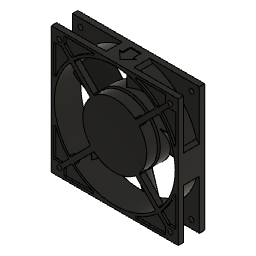
Fan 120mm (Autodesk Fusion 360 design; units mm, degrees)
Autodesk Fusion 360 part; units mm, degrees
sketch "Frame1" plane through (0, 0, 0) normal (0, 1, 0) x (1, 0, 0)
  line L0 (60, 60) -> (-60, 60)
  line L1 (-60, 60) -> (-60, -60)
  line L2 (-60, -60) -> (60, -60)
  line L3 (60, -60) -> (60, 60)
  line L4 (60, 60) -> (-60, -60) construction
  line L5 (-60, 60) -> (60, -60) construction
  circle A0 centre (0, 0) radius 57.125
  circle A1 centre (0, 0) radius 30.25
  circle A2 centre (-52.5, -52.5) radius 2.3
  line L6 (-65, 0) -> (65, 0) construction
  line L7 (0, -65) -> (0, 65) construction
  circle A3 centre (-52.5, 52.5) radius 2.3
  circle A4 centre (52.5, -52.5) radius 2.3
  circle A5 centre (52.5, 52.5) radius 2.3
  circle A6 centre (0, 0) radius 59.4
  line L8 (57.75, -57.75) -> (-57.75, -57.75)
  line L9 (-57.75, -57.75) -> (-57.75, 57.75)
  line L10 (-57.75, 57.75) -> (57.75, 57.75)
  line L11 (57.75, 57.75) -> (57.75, -57.75)
  line L12 (57.75, -57.75) -> (-57.75, 57.75) construction
  line L13 (-57.75, -57.75) -> (57.75, 57.75) construction
  line L14 (-60, -60) -> (-48, -60)
  line L15 (-48, -60) -> (-48, -48)
  line L16 (-48, -48) -> (-60, -48)
  line L17 (-60, -48) -> (-60, -60)
  line L18 (-48, 60) -> (-48, 48)
  line L19 (-48, 48) -> (-60, 48)
  line L20 (48, -60) -> (48, -48)
  line L21 (48, -48) -> (60, -48)
  line L22 (48, 48) -> (60, 48)
  line L23 (48, 60) -> (48, 48)
  line L24 (-9.1263, -5.8737) -> (5.8737, 9.1263) construction
  line L25 (2.5831, -0.6696) -> (-40.3443, -43.597) construction
  line L26 (-40.8339, -38.1469) -> (-47.3531, -44.6661) construction
  line L27 (-38.9044, -41.5914) -> (-49.6566, -52.3436) construction
  line L28 (-44, -38) -> (-38.4801, -43.5199) construction
  line L29 (-42.3435, -39.6565) -> (-39.6565, -42.3435)
  line L30 (-39.6565, -42.3435) -> (-48.8653, -51.5523)
  line L31 (-48.8653, -51.5523) -> (-51.5523, -48.8653)
  line L32 (-51.5523, -48.8653) -> (-42.3435, -39.6565)
  line L33 (-39.6565, 42.3435) -> (-48.8653, 51.5523)
  line L34 (-51.5523, 48.8653) -> (-42.3435, 39.6565)
  line L35 (51.5523, -48.8653) -> (42.3435, -39.6565)
  line L36 (39.6565, -42.3435) -> (48.8653, -51.5523)
  line L37 (51.5523, 48.8653) -> (42.3435, 39.6565)
  line L38 (39.6565, 42.3435) -> (48.8653, 51.5523)
  line L39 (-1.6263, 1.6263) -> (1.6263, -1.6263)
  line L40 (1.6263, -1.6263) -> (-39.0908, -42.3435)
  line L41 (-39.0908, -42.3435) -> (-42.3435, -39.0908)
  line L42 (-42.3435, -39.0908) -> (-1.6263, 1.6263)
  line L43 (1.6263, 1.6263) -> (-39.0908, 42.3435)
  line L44 (-42.3435, 39.0908) -> (-1.6263, -1.6263)
  line L45 (42.3435, 39.0908) -> (1.6263, -1.6263)
  line L46 (-1.6263, 1.6263) -> (39.0908, 42.3435)
  line L47 (42.3435, -39.0908) -> (1.6263, 1.6263)
  line L48 (-1.6263, -1.6263) -> (39.0908, -42.3435)
  dimension "d1" = 120
  dimension "d2" = 120
  dimension "d3" = 114.25
  dimension "d4" = 60.5
  dimension "d5" = 4.6
  dimension "d6" = 7.5
  dimension "d7" = 118.8
  dimension "d8" = 115.5
  dimension "d9" = 115.5
  dimension "d10" = 12
  dimension "d11" = 12
  dimension "d12" = 2.3
  dimension "d13" = 2.3
  dimension "d14" = 1.9
  dimension "d15" = 1.9
  constraint perpendicular L0 L1
  constraint parallel L0 L2
  constraint parallel L1 L3
  constraint horizontal L0
  constraint coincident L4 A0.centre
  constraint coincident L5 A0.centre
  constraint coincident A0.centre A1.centre
  constraint concentric A0 A1
  constraint coincident L4 A2.centre
  constraint perpendicular L3 L6
  constraint perpendicular L0 L7
  constraint symmetric A2 L6 A3
  constraint symmetric A2 L7 A4
  constraint symmetric L7 A3 A5
  constraint perpendicular L8 L9
  constraint parallel L8 L10
  constraint parallel L9 L11
  constraint horizontal L8
  constraint coincident L12 A0.centre
  constraint coincident L13 A0.centre
  constraint horizontal L14
  constraint vertical L15
  constraint horizontal L16
  constraint vertical L17
  constraint symmetric L6 L14.end L18.start
  constraint symmetric L6 L15.end L18.end
  constraint symmetric L6 L16.end L19.end
  constraint symmetric L7 L14.end L20.start
  constraint symmetric L7 L15.end L20.end
  constraint symmetric L7 L16.end L21.end
  constraint symmetric L7 L18.start L23.start
  constraint symmetric L7 L18.end L22.start
  constraint symmetric L7 L19.end L22.end
  constraint perpendicular L12 L24
  constraint coincident A6 L25.end
  constraint parallel L4 L25
  constraint parallel L13 L26
  constraint parallel L13 L27
  constraint perpendicular L25 L28
  constraint perpendicular L29 L30
  constraint parallel L29 L31
  constraint parallel L30 L32
  constraint coincident L28 L29.end
  constraint coincident L27 L29.end
  constraint perpendicular L27 L29
  constraint coincident L26 L29.start
  constraint symmetric L6 L29.start L34.end
  constraint symmetric L6 L29.end L33.start
  constraint symmetric L6 L30.end L33.end
  constraint symmetric L6 L31.end L34.start
  constraint symmetric L7 L29.start L35.end
  constraint symmetric L7 L29.end L36.start
  constraint symmetric L7 L30.end L36.end
  constraint symmetric L7 L31.end L35.start
  constraint symmetric L7 L33.start L38.start
  constraint symmetric L7 L33.end L38.end
  constraint symmetric L7 L34.start L37.start
  constraint symmetric L7 L34.end L37.end
  constraint perpendicular L39 L40
  constraint parallel L39 L41
  constraint parallel L40 L42
  constraint coincident L25 L39.end
  constraint coincident L5 L39.end
  constraint midpoint L24 L39.start
  constraint symmetric L6 L39.start L44.end
  constraint symmetric L6 L39.end L43.start
  constraint symmetric L6 L40.end L43.end
  constraint symmetric L6 L41.end L44.start
  constraint symmetric L7 L39.start L43.start
  constraint symmetric L7 L39.end L44.end
  constraint symmetric L7 L40.end L48.end
  constraint symmetric L7 L41.end L47.start
  constraint symmetric L7 L43.start L39.start
  constraint symmetric L7 L43.end L46.end
  constraint symmetric L7 L44.start L45.start
  constraint symmetric L7 L44.end L39.end
  measures "d1" distance of L1.end L2.end
  measures "d2" distance of L0.end L1.end
  measures "d3" diameter of A0
  measures "d4" diameter of A1
  measures "d5" diameter of A2
  measures "d6" distance of L1 A2.centre
  measures "d7" diameter of A6
  measures "d8" distance of L9.end L10.end
  measures "d9" distance of L8.end L9.end
  measures "d10" distance of L1.end L14.end
  measures "d11" distance of L1.end L16.end
  measures "d12" distance of L4 L24
  measures "d13" distance of L13 L25
  measures "d14" distance of L4 L26
  measures "d15" distance of L4 L27
  measures "d49" diameter of L0.start
extrude "Extrude1" add sketch "Frame1" against normal blind 5 from surface at -7.5 contours L0 L3 L10 L11 L22 L23 | L0 A6 L10 L18 L23 | L3 A6 L11 L21 L22 | L0 L1 L9 L10 L18 L19 | L10 L11 L22 L23 | L2 L3 L8 L11 L20 L21 | L9 L10 L18 L19 | A6 L10 | A6 L8 L9 L10 L11 L29 L30 L32 | A6 L22 L23 L37 L38 | L8 L11 L20 L21 | A6 L11 | L1 A6 L9 L16 L19 | A6 L18 L19 L33 L34 | L2 A6 L8 L15 L20 | A6 L20 L21 L35 L36 | L1 L2 L8 L9 L14 L15 L16 L17 | L8 L9 L15 L16 L30 L31 L32 | A6 L9 | A6 L8 | A6 L15 L16 L30 L32 | L15 L16 L30 L31 L32 | A6 L29 L30 L32 | A0 A1 L45 L46 | A0 A1 L47 L48 | A1 L43 L45 L46 L47 | A1 L45 L47 | A1 L40 L45 L47 L48 | A0 A1 L43 L44 | A1 L43 L46 | L39 L43 L45 L46 L47 | A0 L40 L41 L42 | A0 A1 L40 L42 | A1 L40 L48 | A1 L42 L43 L44 L46 | L39 L40 L42 L44 L48 | A1 L40 L42 L44 L48 | A1 L42 L44 makes body 1
extrude "Extrude2" add sketch "Frame1" along normal blind 5 from surface at 7.5 separate body contours L0 L3 L10 L11 L22 L23 | L0 A6 L10 L18 L23 | L3 A6 L11 L21 L22 | L0 L1 L9 L10 L18 L19 | L10 L11 L22 L23 | L2 L3 L8 L11 L20 L21 | L9 L10 L18 L19 | A6 L10 | A6 L8 L9 L10 L11 L29 L30 L32 | A6 L22 L23 L37 L38 | L8 L11 L20 L21 | A6 L11 | L1 A6 L9 L16 L19 | A6 L18 L19 L33 L34 | L2 A6 L8 L15 L20 | A6 L20 L21 L35 L36 | L1 L2 L8 L9 L14 L15 L16 L17 | L8 L9 L15 L16 L30 L31 L32 | A6 L9 | A6 L8 | A6 L15 L16 L30 L32 | L15 L16 L30 L31 L32 | A6 L29 L30 L32 | A0 L40 L41 L42 makes body 2
fillet "Fillet1" radius 1 32 edges at (13.9031, 10, 57.75) (-13.9031, 10, 57.75) (-48, 10, 57.75) (-48, 10, 50.687) (-40.6371, 10, 43.3242) (48, 10, 57.75) (48, 10, 50.687) (40.6371, 10, 43.3242) (43.3242, 10, 40.6371) (50.687, 10, 48) (57.75, 10, 48) (57.75, 10, 13.9031) (57.75, 10, -13.9031) (43.3242, 10, -40.6371) (50.687, 10, -48) (57.75, 10, -48) (40.6371, 10, -43.3242) (48, 10, -50.687) (48, 10, -57.75) (13.9031, 10, -57.75) (-13.9031, 10, -57.75) (-48, 10, -57.75) (-48, 10, -50.687) (-40.6371, 10, -43.3242) (-43.3242, 10, -40.6371) (-50.687, 10, -48) (-57.75, 10, -48) (-57.75, 10, -13.9031) (-57.75, 10, 13.9031) (-57.75, 10, 48) (-50.687, 10, 48) (-43.3242, 10, 40.6371) on bodies 2
extrude "Extrude3" add sketch "Frame1" against normal blind 3 from surface at -7.5 contours A6 L10 L23 L38 | A6 L11 L22 L37 | A6 L10 L18 L33 | A6 L11 L21 L35 | A6 L9 L19 L34 | A6 L8 L20 L36 | A6 L9 L16 L32 | A6 L8 L15 L30 bodies 1
extrude "Extrude4" add sketch "Frame1" along normal blind 3 from surface at 7.5 contours A6 L10 L23 L38 | A6 L11 L22 L37 | A6 L10 L18 L33 | A6 L11 L21 L35 | A6 L9 L19 L34 | A6 L8 L20 L36 | A6 L9 L16 L32 | A6 L8 L15 L30 bodies 2
extrude "Extrude5" add sketch "Frame1" against normal blind 5 from surface at -2.5 contours A1 L43 L45 L46 L47 | A1 L45 L47 | A1 L40 L45 L47 L48 | A1 L43 L46 | L39 L43 L45 L46 L47 | A1 L40 L48 | A1 L42 L43 L44 L46 | L39 L40 L42 L44 L48 | A1 L40 L42 L44 L48 | A1 L42 L44 bodies 1
fillet "Fillet2" radius 1 52 edges at (13.9031, -11.5, 57.75) (48, -11.5, 57.75) (40.6371, -11.5, 43.3242) (48, -11.5, 50.687) (43.3242, -11.5, 40.6371) (50.687, -11.5, 48) (57.75, -11.5, 48) (57.75, -11.5, 13.9031) (57.75, -11.5, -13.9031) (43.3242, -11.5, -40.6371) (50.687, -11.5, -48) (57.75, -11.5, -48) (40.6371, -11.5, -43.3242) (48, -11.5, -50.687) (48, -11.5, -57.75) (13.9031, -11.5, -57.75) (-13.9031, -11.5, -57.75) (-48, -11.5, -57.75) (-48, -11.5, -50.687) (-40.6371, -11.5, -43.3242) (-43.3242, -11.5, -40.6371) (-50.687, -11.5, -48) (-57.75, -11.5, -48) (-57.75, -11.5, -13.9031) (-57.75, -11.5, 13.9031) (-43.3242, -11.5, 40.6371) (-50.687, -11.5, 48) (-57.75, -11.5, 48) (-40.6371, -11.5, 43.3242) (-48, -11.5, 50.687) (-48, -11.5, 57.75) (-13.9031, -11.5, 57.75) (38.7344, -10, 41.9871) (19.7017, -10, 22.9544) (22.9544, -10, 19.7017) (41.9871, -10, 38.7344) (-38.7344, -10, 41.9871) (-41.9871, -10, 38.7344) (-22.9544, -10, 19.7017) (-19.7017, -10, 22.9544) (-22.9544, -10, -19.7017) (-19.7017, -10, -22.9544) (-41.9871, -10, -38.7344) (-38.7344, -10, -41.9871) (38.7344, -10, -41.9871) (41.9871, -10, -38.7344) (22.9544, -10, -19.7017) (19.7017, -10, -22.9544) (-21.39, -7.5, -21.39) (-21.39, -7.5, 21.39) (21.39, -7.5, 21.39) (21.39, -7.5, -21.39) on bodies 1
sketch "Frame2" plane through (0, -7.5, 0) normal (0, 1, 0) x (-1, 0, 0)
  line L0 (60, -60) -> (60, 60)
  line L1 (60, 60) -> (-60, 60)
  line L2 (-60, 60) -> (-60, -60)
  line L3 (-60, -60) -> (60, -60)
  circle A0 centre (-52.5, -52.5) radius 2.3
  arc A1 (-23.6635, -20.4108) -> (-20.4108, -23.6635) centre (0, 0) ccw
  line L4 (-23.6635, -20.4108) -> (-41.2441, -37.9914)
  arc A2 (-42.6986, -37.9486) -> (-41.2441, -37.9914) centre (-41.9512, -37.2843) ccw
  arc A3 (-42.6986, 37.9486) -> (-42.6986, -37.9486) centre (0, 0) ccw
  arc A4 (-41.2441, 37.9914) -> (-42.6986, 37.9486) centre (-41.9512, 37.2843) ccw
  line L5 (-41.2441, 37.9914) -> (-23.6635, 20.4108)
  arc A5 (-20.4108, 23.6635) -> (-23.6635, 20.4108) centre (0, 0) ccw
  line L6 (-20.4108, 23.6635) -> (-37.9914, 41.2441)
  arc A6 (-37.9486, 42.6986) -> (-37.9914, 41.2441) centre (-37.2843, 41.9512) ccw
  arc A7 (37.9486, 42.6986) -> (-37.9486, 42.6986) centre (0, 0) ccw
  arc A8 (37.9914, 41.2441) -> (37.9486, 42.6986) centre (37.2843, 41.9512) ccw
  line L7 (37.9914, 41.2441) -> (20.4108, 23.6635)
  arc A9 (23.6635, 20.4108) -> (20.4108, 23.6635) centre (0, 0) ccw
  line L8 (23.6635, 20.4108) -> (41.2441, 37.9914)
  arc A10 (42.6986, 37.9486) -> (41.2441, 37.9914) centre (41.9512, 37.2843) ccw
  arc A11 (42.6986, -37.9486) -> (42.6986, 37.9486) centre (0, 0) ccw
  arc A12 (41.2441, -37.9914) -> (42.6986, -37.9486) centre (41.9512, -37.2843) ccw
  line L9 (41.2441, -37.9914) -> (23.6635, -20.4108)
  arc A13 (20.4108, -23.6635) -> (23.6635, -20.4108) centre (0, 0) ccw
  line L10 (20.4108, -23.6635) -> (37.9914, -41.2441)
  arc A14 (37.9486, -42.6986) -> (37.9914, -41.2441) centre (37.2843, -41.9512) ccw
  arc A15 (-37.9486, -42.6986) -> (37.9486, -42.6986) centre (0, 0) ccw
  arc A16 (-37.9914, -41.2441) -> (-37.9486, -42.6986) centre (-37.2843, -41.9512) ccw
  line L11 (-37.9914, -41.2441) -> (-20.4108, -23.6635)
  circle A17 centre (52.5, 52.5) radius 2.3
  circle A18 centre (52.5, -52.5) radius 2.3
  circle A19 centre (-52.5, 52.5) radius 2.3
  circle A20 centre (0, 0) radius 57.125
  circle A21 centre (0, 0) radius 59.4
  line L12 (-60, -16) -> (-60, 16)
  line L13 (60, 16) -> (60, -16)
  line L14 (60, -16) -> (-60, 16) construction
  line L15 (-60, -16) -> (60, 16) construction
  line L16 (16, 60) -> (-16, 60)
  line L17 (-16, -60) -> (16, -60)
  line L18 (16, 60) -> (-16, -60) construction
  line L19 (-16, 60) -> (16, -60) construction
  line L20 (16, 57.2045) -> (16, 60)
  line L21 (-16, 60) -> (-16, 57.2045)
  line L22 (-16, -57.2045) -> (-16, -60)
  line L23 (57.2045, 16) -> (60, 16)
  line L24 (60, -16) -> (57.2045, -16)
  line L25 (16, -60) -> (16, -57.2045)
  line L26 (-57.2045, -16) -> (-60, -16)
  line L27 (-60, 16) -> (-57.2045, 16)
  dimension "d33" = 114.25
  dimension "d34" = 118.8
  dimension "d35" = 120
  dimension "d36" = 32
  dimension "d37" = 120
  dimension "d38" = 32
  constraint coincident A1.centre A3.centre
  constraint perpendicular L12 L24
  constraint parallel L24 L27
  constraint parallel L12 L13
  constraint horizontal L24
  constraint coincident L14 A1.centre
  constraint coincident L15 A1.centre
  constraint perpendicular L16 L21
  constraint parallel L16 L17
  constraint parallel L21 L25
  constraint horizontal L16
  constraint coincident L18 A1.centre
  constraint coincident L19 A1.centre
  constraint collinear L20 L25
  constraint coincident A21 L20.start
  constraint coincident A21 L21.end
  constraint collinear L21 L22
  constraint collinear L23 L27
  constraint coincident A21 L23.start
  constraint coincident A21 L24.end
  constraint coincident A21 L26.start
  constraint coincident A21 L27.end
  constraint coincident A21 L22.start
  constraint coincident A21 L25.end
  measures "d33" diameter of A20
  measures "d34" diameter of A21
  measures "d35" distance of L12.end L13.start
  measures "d36" distance of L12.start L12.end
  measures "d37" distance of L16.end L17.start
  measures "d38" distance of L17.start L17.end
extrude "Extrude6" add sketch "Frame2" along normal blind 15 separate body contours L0 A21 L13 L23 L24 | L3 A21 L17 L22 L25 | A21 | L1 A21 L16 L20 L21 | L2 A21 L12 L26 L27 makes body 3
chamfer "Chamfer1" distance 2.79 angle 45 8 edges at (-16, 0, 60) (16, 0, 60) (-60, 0, 16) (-60, 0, -16) (60, 0, 16) (60, 0, -16) (16, 0, -60) (-16, 0, -60) on bodies 3
combine "Combine1" operation add target body 1 tool bodies 2 3
sketch "Motor" plane through (0, 12.5, 0) normal (0, 1, 0) x (-1, 0, 0)
  line L0 (-50.3941, 47.7071) -> (-44.0035, 41.3165)
  arc A0 (-43.9704, 39.937) -> (-44.0035, 41.3165) centre (-44.7106, 40.6094) ccw
  arc A1 (-43.9704, 39.937) -> (-55.8104, 20.3361) centre (0, 0) ccw
  arc A2 (-57.75, 20.6784) -> (-55.8104, 20.3361) centre (-56.75, 20.6784) ccw
  line L1 (-57.75, 20.6784) -> (-57.75, 47)
  arc A3 (-56.75, 48) -> (-57.75, 47) centre (-56.75, 47) ccw
  line L2 (-56.75, 48) -> (-51.1012, 48)
  arc A4 (-50.3941, 47.7071) -> (-51.1012, 48) centre (-51.1012, 47) ccw
  circle A5 centre (0, 0) radius 57.125
  line L3 (-48, 51.1012) -> (-48, 56.75)
  arc A6 (-47, 57.75) -> (-48, 56.75) centre (-47, 56.75) ccw
  line L4 (-47, 57.75) -> (-20.6784, 57.75)
  arc A7 (-20.3361, 55.8104) -> (-20.6784, 57.75) centre (-20.6784, 56.75) ccw
  arc A8 (-20.3361, 55.8104) -> (-39.937, 43.9704) centre (0, 0) ccw
  arc A9 (-41.3165, 44.0035) -> (-39.937, 43.9704) centre (-40.6094, 44.7106) ccw
  line L5 (-41.3165, 44.0035) -> (-47.7071, 50.3941)
  arc A10 (-48, 51.1012) -> (-47.7071, 50.3941) centre (-47, 51.1012) ccw
  line L6 (44.0035, 41.3165) -> (50.3941, 47.7071)
  arc A11 (51.1012, 48) -> (50.3941, 47.7071) centre (51.1012, 47) ccw
  line L7 (51.1012, 48) -> (56.75, 48)
  arc A12 (57.75, 47) -> (56.75, 48) centre (56.75, 47) ccw
  line L8 (57.75, 47) -> (57.75, 20.6784)
  arc A13 (55.8104, 20.3361) -> (57.75, 20.6784) centre (56.75, 20.6784) ccw
  arc A14 (55.8104, 20.3361) -> (43.9704, 39.937) centre (0, 0) ccw
  arc A15 (44.0035, 41.3165) -> (43.9704, 39.937) centre (44.7106, 40.6094) ccw
  line L9 (48, -51.1012) -> (48, -56.75)
  arc A16 (47, -57.75) -> (48, -56.75) centre (47, -56.75) ccw
  line L10 (47, -57.75) -> (20.6784, -57.75)
  arc A17 (20.3361, -55.8104) -> (20.6784, -57.75) centre (20.6784, -56.75) ccw
  arc A18 (20.3361, -55.8104) -> (39.937, -43.9704) centre (0, 0) ccw
  arc A19 (41.3165, -44.0035) -> (39.937, -43.9704) centre (40.6094, -44.7106) ccw
  line L11 (41.3165, -44.0035) -> (47.7071, -50.3941)
  arc A20 (48, -51.1012) -> (47.7071, -50.3941) centre (47, -51.1012) ccw
  line L12 (50.3941, -47.7071) -> (44.0035, -41.3165)
  arc A21 (43.9704, -39.937) -> (44.0035, -41.3165) centre (44.7106, -40.6094) ccw
  arc A22 (43.9704, -39.937) -> (55.8104, -20.3361) centre (0, 0) ccw
  arc A23 (57.75, -20.6784) -> (55.8104, -20.3361) centre (56.75, -20.6784) ccw
  line L13 (57.75, -20.6784) -> (57.75, -47)
  arc A24 (56.75, -48) -> (57.75, -47) centre (56.75, -47) ccw
  line L14 (56.75, -48) -> (51.1012, -48)
  arc A25 (50.3941, -47.7071) -> (51.1012, -48) centre (51.1012, -47) ccw
  line L15 (47.7071, 50.3941) -> (41.3165, 44.0035)
  arc A26 (39.937, 43.9704) -> (41.3165, 44.0035) centre (40.6094, 44.7106) ccw
  arc A27 (39.937, 43.9704) -> (20.3361, 55.8104) centre (0, 0) ccw
  arc A28 (20.6784, 57.75) -> (20.3361, 55.8104) centre (20.6784, 56.75) ccw
  line L16 (20.6784, 57.75) -> (47, 57.75)
  arc A29 (48, 56.75) -> (47, 57.75) centre (47, 56.75) ccw
  line L17 (48, 56.75) -> (48, 51.1012)
  arc A30 (47.7071, 50.3941) -> (48, 51.1012) centre (47, 51.1012) ccw
  line L18 (-47.7071, -50.3941) -> (-41.3165, -44.0035)
  arc A31 (-39.937, -43.9704) -> (-41.3165, -44.0035) centre (-40.6094, -44.7106) ccw
  arc A32 (-39.937, -43.9704) -> (-20.3361, -55.8104) centre (0, 0) ccw
  arc A33 (-20.6784, -57.75) -> (-20.3361, -55.8104) centre (-20.6784, -56.75) ccw
  line L19 (-20.6784, -57.75) -> (-47, -57.75)
  arc A34 (-48, -56.75) -> (-47, -57.75) centre (-47, -56.75) ccw
  line L20 (-48, -56.75) -> (-48, -51.1012)
  arc A35 (-47.7071, -50.3941) -> (-48, -51.1012) centre (-47, -51.1012) ccw
  line L21 (-44.0035, -41.3165) -> (-50.3941, -47.7071)
  arc A36 (-51.1012, -48) -> (-50.3941, -47.7071) centre (-51.1012, -47) ccw
  line L22 (-51.1012, -48) -> (-56.75, -48)
  arc A37 (-57.75, -47) -> (-56.75, -48) centre (-56.75, -47) ccw
  line L23 (-57.75, -47) -> (-57.75, -20.6784)
  arc A38 (-55.8104, -20.3361) -> (-57.75, -20.6784) centre (-56.75, -20.6784) ccw
  arc A39 (-55.8104, -20.3361) -> (-43.9704, -39.937) centre (0, 0) ccw
  arc A40 (-44.0035, -41.3165) -> (-43.9704, -39.937) centre (-44.7106, -40.6094) ccw
  circle A41 centre (-52.5, -52.5) radius 2.3
  circle A42 centre (-52.5, 52.5) radius 2.3
  circle A43 centre (52.5, -52.5) radius 2.3
  circle A44 centre (52.5, 52.5) radius 2.3
  line L24 (60, -60) -> (60, 60)
  line L25 (60, 60) -> (-60, 60)
  line L26 (-60, 60) -> (-60, -60)
  line L27 (-60, -60) -> (60, -60)
  circle A45 centre (0, 0) radius 31
  dimension "d42" = 62
  constraint concentric A1 A45
  measures "d42" diameter of A45
extrude "Extrude7" add sketch "Motor" against normal blind 12 from surface at -1 separate body contours A45 makes body 4
sketch "Prop1" plane through (0, 0, 0) normal (1, 0, 0) x (0, 1, 0)
  line L0 (-5, 15) -> (20, 15) construction
  line L1 (-5, -15) -> (20, -15) construction
  arc A0 (11.0436, -15) -> (0, 15) centre (-48.7495, -19.9784) ccw
  arc A1 (11.0436, -15) -> (0, 15) centre (-28.8883, -12.6671) ccw
  dimension "d46" = 15
  dimension "d47" = 15
  dimension "d48" = 80
  dimension "d49" = 120
  constraint horizontal L0
  constraint horizontal L1
  constraint coincident L0 A0.end
  constraint coincident L1 A0.start
  measures "d46" vertical distance of origin L0.start
  measures "d47" distance of origin L1
  measures "d48" diameter of A1
  measures "d49" diameter of A0
extrude "Extrude8" add sketch "Prop1" along normal blind 60 separate body makes body 5
sketch "Prop2" plane through (0, 0, 0) normal (0, 1, 0) x (1, 0, 0)
  circle A0 centre (0, 0) radius 55.5
  line L0 (53.4659, -14.8877) -> (53.4659, 130) construction
  circle A1 centre (49.6989, 75.0334) radius 90
  circle A2 centre (49.6989, -75.0334) radius 90
  dimension "d52" = 111
  dimension "d53" = 180
  dimension "d54" = 180
  constraint coincident A0.centre origin
  constraint coincident A0 L0.start
  constraint vertical L0
  constraint coincident L0.start A1
  constraint coincident A0.centre A1
  constraint coincident A0.centre A2
  measures "d52" diameter of A0
  measures "d53" diameter of A1
  measures "d54" diameter of A2
extrude "Extrude9" cut sketch "Prop2" along normal blind 20 contours A0 A1 A2 picked at (46.6279, 0) keep common part bodies 5
copy_body "CopyPasteBodies1" bodies 5 makes body 6
copy_body "CopyPasteBodies2" bodies 6 makes body 7
move_body "Move1" bodies 7 to x (0.309017, 0, 0.951057) y (0, 1, 0) z (-0.951057, 0, 0.309017) at (0, 0, 0)
move_body "Move2" bodies 6 to x (-0.809017, 0, 0.587785) y (0, 1, 0) z (-0.587785, 0, -0.809017) at (0, 0, 0)
copy_body "CopyPasteBodies3" bodies 6 makes body 8
move_body "Move3" bodies 8 to x (0.309017, 0, 0.951057) y (0, 1, 0) z (-0.951057, 0, 0.309017) at (0, 0, 0)
copy_body "CopyPasteBodies4" bodies 8 makes body 9
move_body "Move4" bodies 9 to x (0.309017, 0, 0.951057) y (0, 1, 0) z (-0.951057, 0, 0.309017) at (0, 0, 0)
combine "Combine2" operation add target body 4 tool bodies 5 8 9 7 6
sketch "Arrow" plane through (0, 0, 60) normal (0, 0, 1) x (-1, 0, 0)
  line L0 (13.21, 7.5) -> (60, 7.5)
  line L1 (60, 7.5) -> (60, 12.5)
  line L2 (60, 12.5) -> (-60, 12.5)
  line L3 (-60, 12.5) -> (-60, 7.5)
  line L4 (-60, 7.5) -> (-13.21, 7.5)
  line L5 (-13.21, 7.5) -> (-13.21, -7.5)
  line L6 (-13.21, -7.5) -> (-60, -7.5)
  line L7 (-60, -7.5) -> (-60, -12.5)
  line L8 (-60, -12.5) -> (60, -12.5)
  line L9 (60, -12.5) -> (60, -7.5)
  line L10 (60, -7.5) -> (13.21, -7.5)
  line L11 (13.21, -7.5) -> (13.21, 7.5)
  line L12 (13.21, -7.5) -> (-13.21, -7.5) construction
  line L13 (13.21, 7.5) -> (-13.21, 7.5) construction
  line L14 (5, -7.5) -> (-5, -7.5)
  line L15 (-5, -7.5) -> (-5, 0)
  line L16 (5, 0) -> (5, -7.5)
  line L17 (-5, 0) -> (-8, 0)
  line L18 (5, 0) -> (8, 0)
  line L19 (8, 0) -> (0, 7.5)
  line L20 (0, 7.5) -> (-8, 0)
  dimension "d61" = 10
  dimension "d62" = 5
  dimension "d63" = 3
  dimension "d64" = 3
  constraint coincident L10.end L11.start
  constraint coincident L5.end L6.start
  constraint coincident L0.start L11.end
  constraint coincident L4.end L5.start
  constraint horizontal L14
  constraint vertical L15
  constraint vertical L16
  constraint coincident L12 L14.start
  constraint perpendicular L15 L17
  constraint perpendicular L16 L18
  constraint midpoint L13 L19.end
  measures "d61" distance of L14.start L14.end
  measures "d62" distance of origin L16
  measures "d63" distance of L15.end L17.end
  measures "d64" distance of L16.start L18.end
extrude "Extrude10" cut sketch "Arrow" against normal blind 1 contours L14 L15 L16 L17 L18 L19 L20 bodies 1
equation "d13 = d12"
equation "d15 = d14"
equation "d33 = d3"
equation "d34 = d7"
equation "d47 = d46"
equation "d62 = d61 / 2"
equation "d64 = d63"
named bodies: "Frame", "Prop", "Blade 1", "Blade 3", "Blade 1 (1)", "Blade 2", "Blade 4", "Blade 5"
